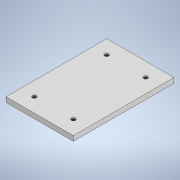
# Autodesk Inventor part: Thermal_underplate
Saved by Autodesk Inventor 2020 (Build 240168000, 168)
## iProperties
Created: 2021-08-09
Part Number: Thermal_underplate
Material: Generic
Document SubType Name: Modeling
Designer: pab2
Density: 1 g/cm^3
Appearance: Default
Author: pab2
Autodesk Inventor part; units mm, degrees
ref_plane "YZ Plane" through (0, 0, 0) normal (1, 0, 0) x (0, 1, 0)
ref_plane "XZ Plane" through (0, 0, 0) normal (0, 1, 0) x (-1, 0, 0)
ref_plane "XY Plane" through (0, 0, 0) normal (0, 0, 1) x (1, 0, 0)
sketch "Sketch1" plane through (0, 0, 0) normal (0, 1, 0) x (-1, 0, 0)
  line L0 (0, 0) -> (85.48, 0)
  line L1 (85.48, 0) -> (85.48, -127.76)
  line L2 (85.48, -127.76) -> (0, -127.76)
  line L3 (0, -127.76) -> (0, 0)
  line L4 (85.48, 0) -> (67.5195, -17.9605)
  line L5 (85.48, 0) -> (110.88, 0) construction
  line L6 (0, 0) -> (17.9605, -17.9605)
  line L7 (85.48, -127.76) -> (67.5195, -109.7995)
  line L8 (85.48, -127.76) -> (110.88, -127.76) construction
  line L9 (0, -127.76) -> (17.9605, -109.7995)
  line L10 (0, -127.76) -> (25.4, -127.76) construction
  dimension "d0" = 85.48
  dimension "d1" = 127.76
  dimension "d2" = 25.4
  dimension "d3" = 135
  dimension "d4" = 25.4
  dimension "d5" = 25.4
  dimension "d6" = 135
  dimension "d7" = 25.4
  dimension "d8" = 45
  constraints: 22 end point, 4 horizontal, 3 equal length, 2 parallel, 1 perpendicular
  measures "d0" distance of L1.end L2.end
  measures "d1" distance of L0.end L1.end
  measures "d2" distance of L0.end L4.end
  measures "d3" angle of L4 L5
  measures "d4" distance of L0.start L6.end
  measures "d5" distance of L1.end L7.end
  measures "d6" angle of L8 L7
  measures "d7" distance of L2.end L9.end
  measures "d8" angle of L10 L9
extrude "Extrusion1" add sketch "Sketch1" along normal blind 6.35
sketch "Sketch2" plane through (0, 0, 0) normal (0, -1, 0) x (1, 0, 0)
  line L0 (-85.48, 0) -> (0, 0) projected
  line L1 (0, 0) -> (-17.9605, -17.9605)
  line L2 (0, 0) -> (25.4, 0) construction
  line L3 (0, 0) -> (0, -127.76) projected
  line L4 (0, -127.76) -> (-17.9605, -109.7995)
  line L5 (0, -127.76) -> (25.4, -127.76) construction
  line L6 (-85.48, -127.76) -> (-85.48, 0) projected
  line L7 (-85.48, 0) -> (-67.5195, -17.9605)
  line L8 (-85.48, 0) -> (-60.08, 0) construction
  line L9 (0, -127.76) -> (-85.48, -127.76) projected
  line L10 (-85.48, -127.76) -> (-67.5195, -109.7995)
  line L11 (-85.48, -127.76) -> (-60.08, -127.76) construction
  dimension "d11" = 25.4
  dimension "d12" = 135
  dimension "d13" = 25.4
  dimension "d14" = 135
  dimension "d15" = 25.4
  dimension "d16" = 45
  dimension "d17" = 25.4
  dimension "d18" = 45
  constraints: 16 end point, 4 equal length, 4 horizontal
  measures "d11" distance of L0.end L1.end
  measures "d12" angle of L1 L2
  measures "d13" distance of L3.end L4.end
  measures "d14" angle of L5 L4
  measures "d15" distance of L0.start L7.end
  measures "d16" angle of L7 L8
  measures "d17" distance of L6.start L10.end
  measures "d18" angle of L11 L10
hole "Hole1" at (-17.9605, 0, -17.9605) at (-67.5195, 0, -17.9605) at (-67.5195, 0, -109.7995) at (-17.9605, 0, -109.7995) direction (0, 1, 0) diameter 5.1054 end through all counterbore diameter 9.525 counterbore depth 4.826 clearance for "Socket Head Cap Screw" size "#10" standard "Ansi Unified Screw Threads"
body "Solid1"
